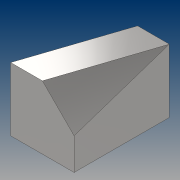
# Autodesk Inventor part: 14
Saved by Autodesk Inventor 2020.2 (Build 242310000, 310)
## iProperties
Created: 2020-09-17
Part Number: 14
Material: 鋼、碳鋼
Document SubType Name: Modeling
Designer: user
Density: 7.85 g/cm^3
Appearance: 半拋光
Mass: 690.8 g
Surface Area: 117.436 cm^2
Volume: 88 cm^3
Author: user
Autodesk Inventor part; units mm, degrees
ref_plane "YZ Plane" through (0, 0, 0) normal (1, 0, 0) x (0, 1, 0)
ref_plane "XZ Plane" through (0, 0, 0) normal (0, 1, 0) x (-1, 0, 0)
ref_plane "XY Plane" through (0, 0, 0) normal (0, 0, 1) x (1, 0, 0)
sketch "草圖1" plane through (0, 0, 0) normal (0, 1, 0) x (-1, 0, 0)
  line L0 (-30, 20) -> (30, 20)
  line L1 (30, 20) -> (30, -20)
  line L2 (30, -20) -> (-30, -20)
  line L3 (-30, -20) -> (-30, 20)
  line L4 (-30, 20) -> (30, -20) construction
  line L5 (30, 20) -> (-30, -20) construction
  point P0 (0, 0)
  dimension "d0" = 40
  dimension "d1" = 60
  constraints: 12 end point, 2 midpoint, 2 parallel, 1 horizontal, 1 perpendicular
  measures "d0" distance of L2.end L0.start
  measures "d1" distance of L1.end L2.end
extrude "擠出1" add sketch "草圖1" along normal blind 40
sketch "草圖2" plane through (-30, 0, -20) normal (-1, 0, 0) x (0, 0, 1)
  line L0 (40, 40) -> (0, 40) construction
  line L1 (20, 40) -> (40, 20)
  line L2 (40, 20) -> (40, 40)
  line L3 (40, 40) -> (20, 40)
  point P0 (20, 0)
  dimension "d4" = 20
  constraints: 6 end point, 2 midpoint, 1 perpendicular, 1 point on line
  measures "d4" distance of L0.start L1.end
loft "斷面混成1" cut profiles "草圖2" section 2 point at (30, 40, 20)
sketch "草圖4" plane through (30, 0, 20) normal (1, 0, 0) x (0, 0, -1)
  line L0 (0, 40) -> (40, 40) construction
  line L1 (40, 40) -> (40, 0) construction
  line L2 (40, 0) -> (0, 0) construction
  line L3 (0, 0) -> (0, 40) construction
  line L4 (0, 20) -> (20, 40) construction
  line L5 (20, 40) -> (40, 20)
  line L6 (40, 0) -> (40, 40) construction
  line L7 (40, 20) -> (40, 40)
  line L8 (40, 40) -> (20, 40) projected
  line L9 (40, 40) -> (20, 40)
  point P0 (20, 0)
  dimension "d9" = 20
  constraints: 6 end point, 2 collinear, 1 midpoint
  measures "d9" distance from line of L0 L5.end
loft "斷面混成2" cut profiles "草圖4" section 2 point at (-30, 40, -20)
